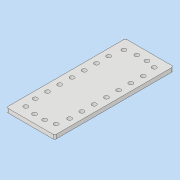
# Autodesk Inventor part: TopCover
Saved by Autodesk Inventor 2018 (Build 220112000, 112)
## iProperties
Created: 2019-08-15
Part Number: TopCover
Material: ABS Plastic
Document SubType Name: Modeling
Designer: Derek Wider
Density: 1.06 g/cm^3
Appearance: Smooth - White
Author: Derek Wider
Autodesk Inventor part; units mm, degrees
ref_plane "YZ Plane" through (0, 0, 0) normal (1, 0, 0) x (0, 1, 0)
ref_plane "XZ Plane" through (0, 0, 0) normal (0, 1, 0) x (-1, 0, 0)
ref_plane "XY Plane" through (0, 0, 0) normal (0, 0, 1) x (1, 0, 0)
sketch "Sketch1" plane through (0, 0, 0) normal (0, 1, 0) x (-1, 0, 0)
  line L0 (0, 0) -> (38.1, 0)
  line L1 (38.1, 0) -> (38.1, -93.98)
  line L2 (38.1, -93.98) -> (0, -93.98)
  line L3 (0, -93.98) -> (0, 0)
  dimension "d0" = 93.98
  dimension "d1" = 38.1
  constraints: 8 end point, 2 parallel, 1 horizontal, 1 perpendicular
  measures "d0" distance of L2.end L0.start
  measures "d1" distance of L1.end L2.end
extrude "Extrusion1" add sketch "Sketch1" along normal blind 3.175
sketch "Sketch2" plane through (0, 3.175, 0) normal (0, 1, 0) x (1, 0, 0)
  circle A0 centre (-7.112, 8.255) radius 1.7145
  line L0 (-38.1, 0) -> (0, 0) projected
  line L1 (0, 0) -> (0, 93.98) projected
  circle A1 centre (-30.988, 8.255) radius 1.7145
  circle A2 centre (-7.112, 85.725) radius 1.7145
  circle A3 centre (-30.988, 85.725) radius 1.7145
  circle A4 centre (-14.4272, 6.604) radius 1.7145
  circle A5 centre (-22.4028, 6.604) radius 1.7145
  circle A6 centre (-14.4272, 87.376) radius 1.7145
  circle A7 centre (-22.4028, 87.376) radius 1.7145
  circle A8 centre (-5.461, 17.3482) radius 1.7145
  circle A9 centre (-5.461, 27.0256) radius 1.7145
  circle A10 centre (-5.461, 36.703) radius 1.7145
  circle A11 centre (-5.461, 46.3804) radius 1.7145
  circle A12 centre (-5.461, 56.0578) radius 1.7145
  circle A13 centre (-5.461, 65.7352) radius 1.7145
  circle A14 centre (-5.461, 75.4126) radius 1.7145
  circle A15 centre (-32.639, 17.3482) radius 1.7145
  circle A16 centre (-32.639, 27.0256) radius 1.7145
  circle A17 centre (-32.639, 36.703) radius 1.7145
  circle A18 centre (-32.639, 46.3804) radius 1.7145
  circle A19 centre (-32.639, 56.0578) radius 1.7145
  circle A20 centre (-32.639, 65.7352) radius 1.7145
  circle A21 centre (-32.639, 75.4126) radius 1.7145
  dimension "d4" = 3.429
  dimension "d5" = 8.255
  dimension "d6" = 7.112
  dimension "d9" = 23.876
  dimension "d12" = 77.47
  dimension "d15" = 14.4272
  dimension "d16" = 6.604
  dimension "d19" = 7.9756
  dimension "d22" = 80.772
  dimension "d25" = 5.461
  dimension "d26" = 17.3482
  dimension "d29" = 9.6774
  dimension "d32" = 27.178
  constraints: 22 centre point, 3 horizontal, 3 vertical, 2 equal radius, 38 other
  measures "d4" diameter of A0
  measures "d5" distance from line of L0 A0.centre
  measures "d6" distance from line of L1 A0.centre
  measures "d9" distance of A0.centre A1.centre
  measures "d12" distance of A0.centre A2.centre
  measures "d15" distance from line of A4.centre L1
  measures "d16" distance from line of L0 A4.centre
  measures "d19" distance of A4.centre A5.centre
  measures "d22" distance of A4.centre A6.centre
  measures "d25" distance from line of A8.centre L1
  measures "d26" distance from line of L0 A8.centre
  measures "d29" distance of A8.centre A9.centre
  measures "d32" distance of A8.centre A15.centre
extrude "Extrusion2" cut sketch "Sketch2" against normal through all
sketch "Sketch3" plane through (0, 0, 0) normal (0, -1, 0) x (1, 0, 0)
  line L0 (-2.54, -3.556) -> (-35.56, -3.556)
  line L1 (-35.56, -3.556) -> (-35.56, -90.424)
  line L2 (-35.56, -90.424) -> (-2.54, -90.424)
  line L3 (-2.54, -90.424) -> (-2.54, -3.556)
  circle A0 centre (-14.4272, -87.376) radius 1.7145 construction
  circle A1 centre (-5.461, -75.4126) radius 1.7145 construction
  line L4 (-38.1, -93.98) -> (0, -93.98) construction
  circle A2 centre (-14.4272, -6.604) radius 1.7145 construction
  point P0 (0, 0)
  point P1 (-19.05, -90.424)
  point P2 (-19.05, -93.98)
  dimension "d37" = 33.02
  dimension "d38" = 3.048
  dimension "d39" = 3.048
  constraints: 8 end point, 2 midpoint, 2 parallel, 1 horizontal, 1 perpendicular, 1 vertical alignment
  measures "d37" distance of L1.end L2.end
  measures "d38" distance from line of L2 A0.centre
  measures "d39" distance from line of L0 A2.centre
extrude "Extrusion3" add sketch "Sketch3" along normal blind 1.016
fillet "Fillet1" radius 1.27 4 edges at (-35.56, -0.508, -3.556) (-35.56, -0.508, -90.424) (-2.54, -0.508, -90.424) (-2.54, -0.508, -3.556)
sketch "Sketch4" plane through (0, 0, 0) normal (0, -1, 0) x (1, 0, 0)
  arc A0 (-2.54, -4.826) -> (-3.81, -3.556) centre (-3.81, -4.826) ccw projected
  line L0 (-3.81, -3.556) -> (-34.29, -3.556) projected
  arc A1 (-34.29, -3.556) -> (-35.56, -4.826) centre (-34.29, -4.826) ccw projected
  line L1 (-35.56, -4.826) -> (-35.56, -89.154) projected
  arc A2 (-35.56, -89.154) -> (-34.29, -90.424) centre (-34.29, -89.154) ccw projected
  line L2 (-34.29, -90.424) -> (-3.81, -90.424) projected
  arc A3 (-3.81, -90.424) -> (-2.54, -89.154) centre (-3.81, -89.154) ccw projected
  line L3 (-2.54, -89.154) -> (-2.54, -4.826) projected
  arc A4 (-0.508, -4.826) -> (-3.81, -1.524) centre (-3.81, -4.826) ccw
  line L4 (-3.81, -1.524) -> (-34.29, -1.524)
  arc A5 (-34.29, -1.524) -> (-37.592, -4.826) centre (-34.29, -4.826) ccw
  line L5 (-37.592, -4.826) -> (-37.592, -89.154)
  arc A6 (-37.592, -89.154) -> (-34.29, -92.456) centre (-34.29, -89.154) ccw
  line L6 (-34.29, -92.456) -> (-3.81, -92.456)
  arc A7 (-3.81, -92.456) -> (-0.508, -89.154) centre (-3.81, -89.154) ccw
  line L7 (-0.508, -89.154) -> (-0.508, -4.826)
  point P0 (0, 0)
  dimension "d43" = 2.032
  constraints: 8 end point, 8 point on circle, 4 centre point, 7 other
  measures "d43" distance between parallel lines of L3 L7
extrude "Extrusion4" cut sketch "Sketch4" against normal blind 1.27
fillet "Fillet2" radius 1.27 4 edges at (-38.1, 1.5875, -93.98) (0, 1.5875, -93.98) (-38.1, 1.5875, 0) (0, 1.5875, 0)
sketch "Sketch5" plane through (0, 3.175, 0) normal (0, 1, 0) x (1, 0, 0)
  arc A0 (-1.27, 0) -> (0, 1.27) centre (-1.27, 1.27) ccw projected
  line L0 (0, 1.27) -> (0, 92.71) projected
  arc A1 (0, 92.71) -> (-1.27, 93.98) centre (-1.27, 92.71) ccw projected
  line L1 (-1.27, 93.98) -> (-36.83, 93.98) projected
  arc A2 (-36.83, 93.98) -> (-38.1, 92.71) centre (-36.83, 92.71) ccw projected
  line L2 (-38.1, 92.71) -> (-38.1, 1.27) projected
  arc A3 (-38.1, 1.27) -> (-36.83, 0) centre (-36.83, 1.27) ccw projected
  line L3 (-36.83, 0) -> (-1.27, 0) projected
  circle A4 centre (-32.639, 65.7352) radius 1.7145 projected
  circle A5 centre (-32.639, 46.3804) radius 1.7145 projected
  circle A6 centre (-32.639, 27.0256) radius 1.7145 projected
  circle A7 centre (-5.461, 75.4126) radius 1.7145 projected
  circle A8 centre (-5.461, 56.0578) radius 1.7145 projected
  circle A9 centre (-5.461, 36.703) radius 1.7145 projected
  circle A10 centre (-5.461, 17.3482) radius 1.7145 projected
  circle A11 centre (-14.4272, 87.376) radius 1.7145 projected
  circle A12 centre (-14.4272, 6.604) radius 1.7145 projected
  circle A13 centre (-7.112, 85.725) radius 1.7145 projected
  circle A14 centre (-7.112, 8.255) radius 1.7145 projected
  circle A15 centre (-30.988, 8.255) radius 1.7145 projected
  circle A16 centre (-30.988, 85.725) radius 1.7145 projected
  circle A17 centre (-22.4028, 6.604) radius 1.7145 projected
  circle A18 centre (-22.4028, 87.376) radius 1.7145 projected
  circle A19 centre (-5.461, 27.0256) radius 1.7145 projected
  circle A20 centre (-5.461, 46.3804) radius 1.7145 projected
  circle A21 centre (-5.461, 65.7352) radius 1.7145 projected
  circle A22 centre (-32.639, 17.3482) radius 1.7145 projected
  circle A23 centre (-32.639, 36.703) radius 1.7145 projected
  circle A24 centre (-32.639, 56.0578) radius 1.7145 projected
  circle A25 centre (-32.639, 75.4126) radius 1.7145 projected
  point P0 (0, 0)
extrude "Extrusion5" cut sketch "Sketch5" against normal through all contours A4 | A5 | A6 | A7 | A8 | A9 | A10 | A11 | A12 | A13 | A14 | A15 | A16 | A17 | A18 | A19 | A20 | A21 | A22 | A23 | A24 | A25
equation "\"d39\" = d38"
body "Solid1"
